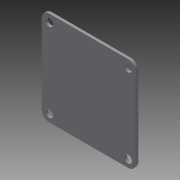
# Autodesk Inventor part: carte
Saved by Autodesk Inventor 2015 (Build 190159000, 159)
## iProperties
Created: 2015-02-16
Part Number: carte
Material: Generic
Document SubType Name: Modeling
Designer: Piotr
Density: 1 g/cm^3
Appearance: Default
Author: Piotr
Autodesk Inventor part; units mm, degrees
ref_plane "YZ Plane" through (0, 0, 0) normal (1, 0, 0) x (0, 1, 0)
ref_plane "XZ Plane" through (0, 0, 0) normal (0, 1, 0) x (-1, 0, 0)
ref_plane "XY Plane" through (0, 0, 0) normal (0, 0, 1) x (1, 0, 0)
sketch "Sketch1" plane through (0, 0, 0) normal (0, 0, 1) x (1, 0, 0)
  line L0 (-12.1557, 15.1728) -> (18.8443, 15.1728)
  line L1 (21.8443, 12.1728) -> (21.8443, -18.8272)
  line L2 (18.8443, -21.8272) -> (-12.1557, -21.8272)
  line L3 (-15.1557, -18.8272) -> (-15.1557, 12.1728)
  arc A0 (-12.1557, 15.1728) -> (-15.1557, 12.1728) centre (-12.1557, 12.1728) ccw
  arc A1 (21.8443, 12.1728) -> (18.8443, 15.1728) centre (18.8443, 12.1728) ccw
  arc A2 (18.8443, -21.8272) -> (21.8443, -18.8272) centre (18.8443, -18.8272) ccw
  arc A3 (-15.1557, -18.8272) -> (-12.1557, -21.8272) centre (-12.1557, -18.8272) ccw
  point P0 (0, 0)
  point P1 (-15.1557, 15.1728)
  point P2 (21.8443, -21.8272)
  point P3 (21.8443, 15.1728)
  dimension "d0" = 37
  dimension "d1" = 37
  dimension "d2" = 3
  constraints: 8 end point, 8 point on circle, 8 tangent, 6 point on line, 4 centre point, 3 equal radius, 2 parallel, 1 horizontal, 1 perpendicular
  measures "d0" distance of point (-15.156, 15.173) point (21.844, 15.173)
  measures "d1" distance of point (21.844, 15.173) point (21.844, -21.827)
  measures "d2" radius of A0
extrude "Extrusion1" add sketch "Sketch1" along normal blind 1
sketch "Sketch2" plane through (0, 0, 1) normal (0, 0, 1) x (1, 0, 0)
  circle A0 centre (-12.1557, 12.1728) radius 1.5
  line L0 (18.8443, 15.1728) -> (-12.1557, 15.1728) projected
  line L1 (-15.1557, 12.1728) -> (-15.1557, -18.8272) projected
  line L2 (3.3443, 8.5218) -> (3.3443, -18.2163) construction
  circle A1 centre (18.8443, 12.1728) radius 1.5
  line L3 (-8.842, -3.3272) -> (14.7627, -3.3272) construction
  circle A2 centre (-12.1557, -18.8272) radius 1.5
  circle A3 centre (18.8443, -18.8272) radius 1.5
  point P0 (0, 0)
  dimension "d5" = 3
  dimension "d6" = 3
  dimension "d7" = 3
  constraints: 4 centre point, 4 end point, 3 symmetric about line, 1 horizontal, 1 vertical, 3 other
  measures "d5" distance from line of L0 A0.centre
  measures "d6" distance from line of L1 A0.centre
  measures "d7" diameter of A0
hole "Hole1" at (18.8443, 12.1728, 1) at (18.8443, -18.8272, 1) at (-12.1557, -18.8272, 1) at (-12.1557, 12.1728, 1) direction (0, 0, -1) diameter 3 end through all
equation "\"d1\" = d0"
body "Solid1"
